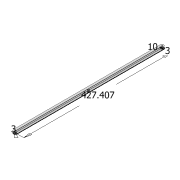
# Autodesk Inventor part: Part_14
Saved by Autodesk Inventor 2022 (Build 260153000, 153)
## iProperties
Created: 2022-04-26
Part Number: Part_14
Material: Generic
Document SubType Name: Modeling
Designer: dell
Density: 1 g/cm^3
Appearance: Default
Author: dell
Autodesk Inventor part; units mm, degrees
ref_plane "YZ Plane" through (0, 0, 0) normal (1, 0, 0) x (0, 1, 0)
ref_plane "XZ Plane" through (0, 0, 0) normal (0, 1, 0) x (-1, 0, 0)
ref_plane "XY Plane" through (0, 0, 0) normal (0, 0, 1) x (1, 0, 0)
sketch "Sketch1" plane through (0, 0, 0) normal (0, 1, 0) x (-1, 0, 0)
  line L0 (0, 0) -> (0, -427.407) construction
  line L1 (-5, 0) -> (-5, -427.407)
  line L2 (5, -427.407) -> (5, 0)
  arc A0 (5, 0) -> (-5, 0) centre (0, 0) ccw
  arc A1 (-5, -427.407) -> (5, -427.407) centre (0, -427.407) ccw
  circle A2 centre (0, 0) radius 1.5
  circle A3 centre (0, -427.407) radius 1.5
  point P0 (0, -213.7035)
  dimension "d1" = 427.407
  dimension "d2" = 10
  dimension "d3" = 3
  dimension "d4" = 3
  constraints: 8 end point, 4 centre point, 4 point on circle, 4 tangent, 2 coincident, 1 midpoint, 1 parallel, 1 vertical
  measures "d1" distance of L0.start L0.end
  measures "d2" diameter of A1
  measures "d3" diameter of A2
  measures "d4" diameter of A3
extrude "Extrusion1" add sketch "Sketch1" along normal blind 6
body "Solid1"
